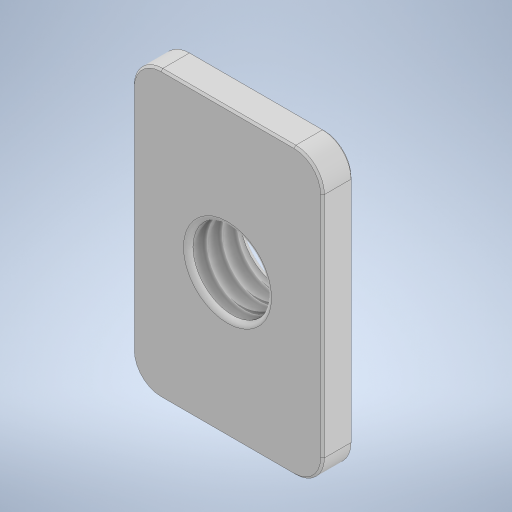
# Autodesk Inventor part: M5 T SLOT NUT
Saved by Autodesk Inventor 2024 (Build 280153000, 153)
## iProperties
Created: 2024-09-05
Part Number: M5 T SLOT NUT
Material: Generic
Document SubType Name: Modeling
Designer: Ishaan
Density: 1 g/cm^3
Appearance: Default
Author: Ishaan
Autodesk Inventor part; units mm, degrees
ref_plane "YZ Plane" through (0, 0, 0) normal (1, 0, 0) x (0, 1, 0)
ref_plane "XZ Plane" through (0, 0, 0) normal (0, 1, 0) x (-1, 0, 0)
ref_plane "XY Plane" through (0, 0, 0) normal (0, 0, 1) x (1, 0, 0)
sketch "Sketch1" plane through (0, 0, 0) normal (0, 0, 1) x (1, 0, 0)
  line L0 (5, -7.5) -> (-5, -7.5)
  line L1 (-5, -7.5) -> (-5, 7.5)
  line L2 (-5, 7.5) -> (5, 7.5)
  line L3 (5, 7.5) -> (5, -7.5)
  line L4 (5, -7.5) -> (-5, 7.5) construction
  line L5 (-5, -7.5) -> (5, 7.5) construction
  point P0 (0, 0)
  dimension "d0" = 10
  dimension "d1" = 15
  constraints: 12 end point, 2 midpoint, 2 parallel, 1 horizontal, 1 perpendicular
  measures "d0" distance of L1.end L2.end
  measures "d1" distance of L0.end L1.end
extrude "Extrusion1" add sketch "Sketch1" against normal blind 1.6
sketch "Sketch2" plane through (0, 0, -1.6) normal (0, 0, -1) x (-1, 0, 0)
  circle A0 centre (0, 0) radius 3.45
  dimension "d4" = 6.9
  constraints: 1 centre point, 1 coincident
  measures "d4" diameter of A0
extrude "Extrusion2" add sketch "Sketch2" along normal blind 1.4
fillet "Fillet1" radius 0.25 1 edges at (3.45, 0, -1.6)
fillet "Fillet2" radius 1.5 4 edges at (5, 7.5, -0.8) (-5, 7.5, -0.8) (-5, -7.5, -0.8) (5, -7.5, -0.8)
sketch "Sketch3" plane through (0, 0, -3) normal (0, 0, -1) x (-1, 0, 0)
  circle A0 centre (0, 0) radius 3.45 projected
  constraints: 1 coincident
hole "Hole1" at (0, 0, -3) direction (0, 0, 1) diameter 4.134 end through all thread size "M5x0.8" class "6H" standard "ANSI Metric M Profile"
fillet "Fillet3" radius 0.25 2 edges at (0, -2.067, 0) (0, -2.067, -3)
chamfer "Chamfer1" distance 0.1 angle 45 1 edges at (3.45, 0, -3)
chamfer "Chamfer2" distance 0.1 angle 45 16 edges at (4.5607, 7.0607, 0) (5, 0, 0) (4.5607, -7.0607, 0) (0, -7.5, 0) (-4.5607, -7.0607, 0) (-5, 0, 0) (-4.5607, 7.0607, 0) (0, 7.5, 0) (4.5607, 7.0607, -1.6) (0, 7.5, -1.6) (-4.5607, 7.0607, -1.6) (-5, 0, -1.6) (-4.5607, -7.0607, -1.6) (0, -7.5, -1.6) (4.5607, -7.0607, -1.6) (5, 0, -1.6)
body "Solid1"
